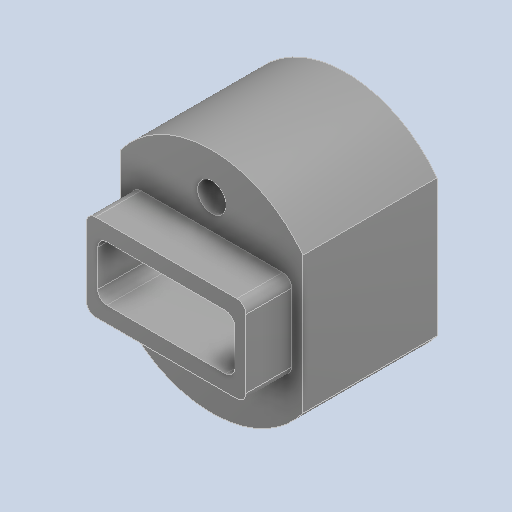
# Autodesk Inventor part: Hip Adapter
Saved by Autodesk Inventor 2022.2 (Build 262287030, 287C)
## iProperties
Created: 2019-10-18
Part Number: Hip Adapter
Material: Generic
Document SubType Name: Modeling
Designer: Jochen
Density: 1 g/cm^3
Appearance: Default
Sending System: SolidWorks 2017
Last Author: Felix
Last Saved: 2021-02-23
Author: Jochen
Autodesk Inventor part; units mm, degrees
ref_plane "YZ Plane" through (0, 0, 0) normal (1, 0, 0) x (0, 1, 0)
ref_plane "XZ Plane" through (0, 0, 0) normal (0, 1, 0) x (-1, 0, 0)
ref_plane "Work Plane1" through (0, 0, -10) normal (0, 0, 1) x (1, 0, 0)
sketch "Sketch1" plane through (0, 0, -10) normal (0, 0, 1) x (1, 0, 0)
  line L0 (0, -17.5) -> (0, 17.5) construction
  line L1 (-14, 0) -> (14, 0) construction
  line L2 (10, -7.5) -> (10, 7.5)
  arc A0 (10, 7.5) -> (-10, 7.5) centre (0, 0) ccw
  line L3 (-10, 7.5) -> (-10, -7.5)
  arc A1 (-10, -7.5) -> (10, -7.5) centre (0, 0) ccw
  circle A2 centre (0, -8) radius 1.55
  circle A3 centre (0, 8) radius 1.55
  line L4 (0, -8) -> (0, 8) construction
  line L5 (-9, -5) -> (9, -5)
  line L6 (9, -5) -> (9, 5)
  line L7 (9, 5) -> (-9, 5)
  line L8 (-9, 5) -> (-9, -5)
  line L9 (-7.5, -3) -> (7.5, -3)
  line L10 (7.5, -3) -> (7.5, 3)
  line L11 (7.5, 3) -> (-7.5, 3)
  line L12 (-7.5, 3) -> (-7.5, -3)
  line L13 (8.75, -4.75) -> (-8.75, -4.75)
  line L14 (-8.75, -4.75) -> (-8.75, 4.75)
  line L15 (-8.75, 4.75) -> (8.75, 4.75)
  line L16 (8.75, 4.75) -> (8.75, -4.75)
  point P0 (0, 0)
  point P1 (-10, 0)
  point P2 (10, 0)
  dimension "d1" = 15
  dimension "d2" = 12.5
  dimension "d3" = 20
  dimension "d4" = 3.1
  dimension "d5" = 16
  dimension "d6" = 18
  dimension "d7" = 10
  dimension "d8" = 15
  dimension "d9" = 6
  dimension "d18" = 0.25
  constraints: 30 end point, 7 parallel, 4 centre point, 4 point on circle, 4 point on line, 3 midpoint, 3 perpendicular, 2 equal radius, 2 horizontal, 1 vertical, 8 other
  measures "d1" distance of L2.start L2.end
  measures "d2" radius of A1
  measures "d3" distance between parallel lines of L3 L2
  measures "d4" diameter of A2
  measures "d5" distance of L4.start L4.end
  measures "d6" distance of L5.start L5.end
  measures "d7" distance of L5.end L6.end
  measures "d8" distance of L9.start L9.end
  measures "d9" distance of L11.end L9.start
  measures "d18" distance between parallel lines of L5 L13
extrude "Extrusion1" add sketch "Sketch1" along normal blind 14.7 contours A1 L3 A0 L2 | L8 L7 L6 L5 | L13 L14 L15 L16
extrude "Extrusion2" add sketch "Sketch1" along normal blind 5 from surface at 14.7 contours L13 L14 L15 L16
extrude "Extrusion3" cut sketch "Sketch1" along normal blind 4.5 contours L8 L7 L6 L5 | L13 L14 L15 L16
fillet "Fillet1" radius 1 12 edges at (-7.5, -3, 2.1) (-7.5, 3, 2.1) (7.5, 3, 2.1) (7.5, -3, 2.1) (9, -5, -7.75) (9, 5, -7.75) (-9, -5, -7.75) (-9, 5, -7.75) (-8.75, -4.75, 7.2) (-8.75, 4.75, 7.2) (8.75, -4.75, 7.2) (8.75, 4.75, 7.2)
chamfer "Chamfer1" distance 0.5 angle 45 8 edges at (9, 0, -10) (8.7071, 4.7071, -10) (0, 5, -10) (-8.7071, 4.7071, -10) (-9, 0, -10) (-8.7071, -4.7071, -10) (0, -5, -10) (8.7071, -4.7071, -10)
body "Solid1"
body "Solid2"
